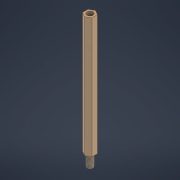
# Autodesk Inventor part: Brass Spacer
Saved by Autodesk Inventor 2022.1 (Build 261234000, 234)
## iProperties
Created: 2021-10-11
Part Number: Brass Spacer
Material: Brass, Soft Yellow
Document SubType Name: Modeling
Designer: Santiago Martínez
Mass: 6.72858 g
Surface Area: 15.9947 cm^2
Volume: 0.794401 cm^3
Density: 8.47 g/cm^3
Appearance: Brindle
Author: Santiago Martínez
Autodesk Inventor part; units mm, degrees
ref_plane "YZ Plane" through (0, 0, 0) normal (1, 0, 0) x (0, 1, 0)
ref_plane "XZ Plane" through (0, 0, 0) normal (0, 1, 0) x (-1, 0, 0)
ref_plane "XY Plane" through (0, 0, 0) normal (0, 0, 1) x (1, 0, 0)
sketch "Sketch1" plane through (0, 0, 0) normal (0, 1, 0) x (-1, 0, 0)
  line L0 (0, -2.7135) -> (-2.35, -1.3568)
  line L1 (-2.35, -1.3568) -> (-2.35, 1.3568)
  line L2 (-2.35, 1.3568) -> (0, 2.7135)
  line L3 (0, 2.7135) -> (2.35, 1.3568)
  line L4 (2.35, 1.3568) -> (2.35, -1.3568)
  line L5 (2.35, -1.3568) -> (0, -2.7135)
  circle A0 centre (0, 0) radius 1.5
  dimension "d1" = 3
  dimension "d4" = 4.7
  constraints: 12 end point, 2 coincident, 1 centre point, 13 other
  measures "d1" diameter of A0
  measures "d4" distance between parallel lines of L1 L4
extrude "Extrusion1" add sketch "Sketch1" along normal blind 60
sketch "Sketch2" plane through (0, 0, 0) normal (0, -1, 0) x (1, 0, 0)
  circle A0 centre (0, 0) radius 1.5 projected
  circle A1 centre (0, 0) radius 1.5
  dimension "d5" = 3
  constraints: 1 centre point, 1 coincident
  measures "d5" diameter of A1
extrude "Extrusion2" add sketch "Sketch2" along normal blind 6 and the other way blind 4
thread "Thread1" size "M3x0.5" class "6g" standard "ANSI Metric M Profile" full length
body "Solid1"
